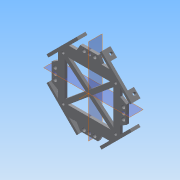
# Autodesk Inventor part: fix_board
Saved by Autodesk Inventor 2015 (Build 190159000, 159)
## iProperties
Created: 2015-06-18
Part Number: fix_board
Material: Générique
Document SubType Name: Modeling
Designer: Gregwar
Density: 1 g/cm^3
Appearance: Par défaut
Author: Gregwar
Autodesk Inventor part; units mm, degrees
ref_plane "YZ Plane" through (0, 0, 0) normal (1, 0, 0) x (0, 1, 0)
ref_plane "XZ Plane" through (0, 0, 0) normal (0, 1, 0) x (-1, 0, 0)
ref_plane "XY Plane" through (0, 0, 0) normal (0, 0, 1) x (1, 0, 0)
sketch "Esquisse1" plane through (0, 0, 0) normal (0, 1, 0) x (-1, 0, 0)
  line L0 (35, 35) -> (35, 14)
  line L1 (35, 14) -> (42, 10)
  line L2 (42, 10) -> (42, 0)
  line L3 (35, 35) -> (0, 0)
  line L4 (42, 0) -> (0, 0) construction
  line L5 (35, -35) -> (35, -14)
  line L6 (35, -14) -> (42, -10)
  line L7 (42, -10) -> (42, 0)
  line L8 (35, -35) -> (0, 0)
  line L9 (38.5, -12) -> (38.5, 12) construction
  circle A0 centre (38.5, 0) radius 2.15
  circle A1 centre (38.5, 6) radius 2.15
  circle A2 centre (38.5, -6) radius 2.15
  dimension "d0" = 90
  dimension "d1" = 70
  dimension "d4" = 6
  dimension "d11" = 6
  dimension "d16" = 4.3
  dimension "d17" = 20
  dimension "d18" = 4
  dimension "d19" = 7
  constraints: 20 end point, 3 centre point, 3 midpoint, 3 symmetric about line, 3 vertical, 1 horizontal, 1 parallel, 4 other
  measures "d0" angle of L3 L8
  measures "d1" distance of L0.start L5.start
  measures "d4" distance of A0.centre A1.centre
  measures "d11" distance of A0.centre A2.centre
  measures "d16" diameter of A0
  measures "d17" distance of L1.end L6.end
  measures "d18" vertical distance of L1.end L0.end
  measures "d19" distance between parallel lines of L5 L7
extrude "Extrusion1" add sketch "Esquisse1" along normal blind 3
pattern_circular "Réseau circulaire1" count 4 over 360 about axis through (0, 0, 0) along (0, 1, 0) of "Extrusion1"
sketch "Esquisse2" plane through (0, 3, 0) normal (0, 1, 0) x (1, 0, 0)
  circle A0 centre (0, -38.5) radius 2.15 construction
  circle A1 centre (6, -38.5) radius 2.15 construction
  circle A2 centre (-6, -38.5) radius 2.15 construction
  circle A3 centre (38.5, -6) radius 2.15 construction
  circle A4 centre (38.5, 6) radius 2.15 construction
  circle A5 centre (38.5, 0) radius 2.15 construction
  circle A6 centre (6, 38.5) radius 2.15 construction
  circle A7 centre (-6, 38.5) radius 2.15 construction
  circle A8 centre (0, 38.5) radius 2.15 construction
  circle A9 centre (-38.5, 6) radius 2.15 construction
  circle A10 centre (-38.5, -6) radius 2.15 construction
  circle A11 centre (-38.5, 0) radius 2.15 construction
  line L0 (-35, 35) -> (-35, 14) construction
  line L1 (-35, 14) -> (-42, 10) construction
  line L2 (-42, 10) -> (-42, -10) construction
  line L3 (-42, -10) -> (-35, -14) construction
  line L4 (-35, -14) -> (-35, -35) construction
  line L5 (-35, -35) -> (-14, -35) construction
  line L6 (-14, -35) -> (-10, -42) construction
  line L7 (-10, -42) -> (10, -42) construction
  line L8 (10, -42) -> (14, -35) construction
  line L9 (14, -35) -> (35, -35) construction
  line L10 (35, -35) -> (35, -14) construction
  line L11 (35, -14) -> (42, -10) construction
  line L12 (42, -10) -> (42, 10) construction
  line L13 (42, 10) -> (35, 14) construction
  line L14 (35, 14) -> (35, 35) construction
  line L15 (35, 35) -> (14, 35) construction
  line L16 (14, 35) -> (10, 42) construction
  line L17 (10, 42) -> (-10, 42) construction
  line L18 (-10, 42) -> (-14, 35) construction
  line L19 (-14, 35) -> (-35, 35) construction
  line L20 (32.5, -27.5) -> (-32.5, -27.5) construction
  line L21 (-32.5, -27.5) -> (-32.5, 27.5) construction
  line L22 (-32.5, 27.5) -> (32.5, 27.5) construction
  line L23 (32.5, 27.5) -> (32.5, -27.5) construction
  line L24 (32.5, -27.5) -> (-32.5, 27.5) construction
  line L25 (-32.5, -27.5) -> (32.5, 27.5) construction
  line L26 (29.5, -24.9615) -> (-29.5, -24.9615) construction
  line L27 (-29.5, -24.9615) -> (-29.5, 24.9615) construction
  line L28 (-29.5, 24.9615) -> (29.5, 24.9615) construction
  line L29 (29.5, 24.9615) -> (29.5, -24.9615) construction
  line L30 (29.5, -24.9615) -> (-29.5, 24.9615) construction
  line L31 (-29.5, -24.9615) -> (29.5, 24.9615) construction
  line L32 (27.5, -23.2692) -> (-27.5, -23.2692)
  line L33 (-27.5, -23.2692) -> (-27.5, 23.2692)
  line L34 (-27.5, 23.2692) -> (27.5, 23.2692)
  line L35 (27.5, 23.2692) -> (27.5, -23.2692)
  line L36 (27.5, -23.2692) -> (-27.5, 23.2692) construction
  line L37 (-27.5, -23.2692) -> (27.5, 23.2692) construction
  circle A12 centre (-29.5, -24.9615) radius 1.65
  circle A13 centre (29.5, -24.9615) radius 1.65
  circle A14 centre (29.5, 24.9615) radius 1.65
  circle A15 centre (-29.5, 24.9615) radius 1.65
  point P0 (0, 0)
  dimension "d25" = 65
  dimension "d26" = 55
  dimension "d27" = 3
  dimension "d28" = 2
  dimension "d29" = 3.3
  constraints: 36 end point, 6 midpoint, 6 parallel, 4 centre point, 4 coincident, 3 equal radius, 3 horizontal, 3 perpendicular, 2 point on line
  measures "d25" distance of L21.end L22.end
  measures "d26" distance of L20.end L21.end
  measures "d27" distance between parallel lines of L21 L27
  measures "d28" distance between parallel lines of L33 L27
  measures "d29" diameter of A12
extrude "Extrusion2" cut sketch "Esquisse2" against normal through all
chamfer "Chanfrein1" distance 8 angle 45 4 edges at (35, 1.5, -35) (-35, 1.5, -35) (-35, 1.5, 35) (35, 1.5, 35)
sketch "Esquisse3" plane through (0, 0, 0) normal (0, -1, 0) x (1, 0, 0)
  circle A0 centre (-29.5, -24.9615) radius 1.65 projected
  circle A1 centre (29.5, 24.9615) radius 1.65 projected
  circle A2 centre (-29.5, 24.9615) radius 1.65 projected
  circle A3 centre (29.5, -24.9615) radius 1.65 projected
  line L0 (27.5, 23.2692) -> (27.5, -23.2692) projected
  line L1 (27.5, -23.2692) -> (-27.5, -23.2692) projected
  line L2 (-27.5, -23.2692) -> (-27.5, 23.2692) projected
  line L3 (-27.5, 23.2692) -> (27.5, 23.2692) projected
  circle A4 centre (0, 38.5) radius 2.15 projected
  circle A5 centre (6, 38.5) radius 2.15 projected
  circle A6 centre (-6, 38.5) radius 2.15 projected
  circle A7 centre (38.5, 6) radius 2.15 projected
  circle A8 centre (38.5, -6) radius 2.15 projected
  circle A9 centre (38.5, 0) radius 2.15 projected
  circle A10 centre (6, -38.5) radius 2.15 projected
  circle A11 centre (-6, -38.5) radius 2.15 projected
  circle A12 centre (0, -38.5) radius 2.15 projected
  circle A13 centre (-38.5, -6) radius 2.15 projected
  circle A14 centre (-38.5, 6) radius 2.15 projected
  circle A15 centre (-38.5, 0) radius 2.15 projected
  line L4 (27, 35) -> (35, 27) projected
  line L5 (27, 35) -> (14, 35) projected
  line L6 (14, 35) -> (10, 42) projected
  line L7 (10, 42) -> (-10, 42) projected
  line L8 (-10, 42) -> (-14, 35) projected
  line L9 (-14, 35) -> (-27, 35) projected
  line L10 (-35, 27) -> (-27, 35) projected
  line L11 (-35, 27) -> (-35, 14) projected
  line L12 (-35, 14) -> (-42, 10) projected
  line L13 (-42, 10) -> (-42, -10) projected
  line L14 (-42, -10) -> (-35, -14) projected
  line L15 (-35, -14) -> (-35, -27) projected
  line L16 (-27, -35) -> (-35, -27) projected
  line L17 (-27, -35) -> (-14, -35) projected
  line L18 (-14, -35) -> (-10, -42) projected
  line L19 (-10, -42) -> (10, -42) projected
  line L20 (10, -42) -> (14, -35) projected
  line L21 (14, -35) -> (27, -35) projected
  line L22 (35, -27) -> (27, -35) projected
  line L23 (35, -27) -> (35, -14) projected
  line L24 (35, -14) -> (42, -10) projected
  line L25 (42, -10) -> (42, 10) projected
  line L26 (42, 10) -> (35, 14) projected
  line L27 (35, 14) -> (35, 27) projected
  line L28 (-47.9706, 14.0294) -> (-14.0294, 47.9706)
  line L29 (-14.0294, 47.9706) -> (-11.9081, 45.8492)
  line L30 (-11.9081, 45.8492) -> (-45.8492, 11.9081)
  line L31 (-45.8492, 11.9081) -> (-47.9706, 14.0294)
  point P0 (0, 0)
  point P1 (-31, 31)
  dimension "d35" = 48
  dimension "d36" = 3
  constraints: 8 end point, 2 midpoint, 2 perpendicular, 1 collinear, 1 parallel
  measures "d35" distance of L28.start L28.end
  measures "d36" distance of L28.end L29.end
extrude "Extrusion3" add sketch "Esquisse3" against normal blind 10 contours L30 L11 L10 L9 | L9 L28 L29 L30 | L30 L31 L28 L11
sketch "Esquisse4" plane through (-14.0294, 0, 47.9706) normal (-0.7071068, 0, 0.7071068) x (0.7071068, 0, 0.7071068)
  line L0 (0, 0) -> (-48, 0) projected
  line L1 (0, 0) -> (0, 10) projected
  line L2 (-48, 10) -> (0, 10) projected
  line L3 (-48, 0) -> (-48, 10) projected
  line L4 (-48, 0) -> (-48, 10) construction
  line L5 (-48, 7) -> (0, 7) construction
  line L6 (0, 0) -> (0, 10) construction
  circle A0 centre (-42.5, 7) radius 1.75
  line L7 (0, 10) -> (-48, 10) construction
  line L8 (-24, 10) -> (-24, 0) construction
  circle A1 centre (-5.5, 7) radius 1.75
  dimension "d41" = 10
  dimension "d42" = 3
  dimension "d43" = 37
  dimension "d44" = 3.5
  constraints: 4 end point, 3 point on line, 2 centre point, 1 horizontal, 1 midpoint, 1 symmetric about line, 1 vertical, 1 other
  measures "d41" distance between parallel lines of L0 L2
  measures "d42" distance between parallel lines of L5 L2
  measures "d43" distance of A0.centre A1.centre
  measures "d44" diameter of A0
extrude "Extrusion4" cut sketch "Esquisse4" against normal through all contours A0 | A1
ref_plane "Plan de construction1" through (0, 0, 14) normal (-1, 0, 0) x (0, 0, 1)
ref_plane "Plan de construction2" through (14, 0, 0) normal (0, 0, -1) x (-1, 0, 0)
sketch "Esquisse6" plane through (-14.0294, 0, 47.9706) normal (-0.7071068, 0, 0.7071068) x (0.7071068, 0, 0.7071068)
  line L0 (-15.3431, 3) -> (-9.1508, 3) projected
  circle A0 centre (-5.5, 7) radius 1.75 projected
  circle A1 centre (-42.5, 7) radius 1.75 projected
  line L1 (0, 0) -> (-48, 0) projected
  line L2 (0, 0) -> (0, 10) projected
  line L3 (-48, 10) -> (0, 10) projected
  line L4 (-48, 0) -> (-48, 10) projected
  line L5 (-10.5, 10) -> (-37.5, 10)
  line L6 (-37.5, 10) -> (-37.5, 3)
  line L7 (-37.5, 3) -> (-10.5, 3)
  line L8 (-10.5, 3) -> (-10.5, 10)
  point P0 (-24, 0)
  point P1 (-24, 10)
  dimension "d51" = 27
  dimension "d63" = 3
  constraints: 8 end point, 2 midpoint, 2 parallel, 1 horizontal, 1 perpendicular
  measures "d51" distance of L6.end L7.end
  measures "d63" distance between parallel lines of L7 L1
extrude "Extrusion5" cut sketch "Esquisse6" against normal through all contours L7 L6 L3 L8 L0
pattern_circular "Réseau circulaire4" count 4 over 360 about axis through (0, 0, 0) along (0, -1, 0) of "Extrusion5", "Extrusion4", "Extrusion3"
sketch "Esquisse8" plane through (0, 0, 0) normal (0, -1, 0) x (1, 0, 0)
  circle A0 centre (-29.5, -24.9615) radius 1.65 construction
  circle A1 centre (29.5, 24.9615) radius 1.65 construction
  circle A2 centre (-29.5, 24.9615) radius 1.65 construction
  circle A3 centre (29.5, -24.9615) radius 1.65 construction
  line L0 (27.5, 23.2692) -> (27.5, -23.2692) construction
  line L1 (27.5, -23.2692) -> (-27.5, -23.2692) construction
  line L2 (-27.5, -23.2692) -> (-27.5, 23.2692) construction
  line L3 (-27.5, 23.2692) -> (27.5, 23.2692) construction
  circle A4 centre (0, 38.5) radius 2.15 construction
  circle A5 centre (6, 38.5) radius 2.15 construction
  circle A6 centre (-6, 38.5) radius 2.15 construction
  circle A7 centre (38.5, 6) radius 2.15 construction
  circle A8 centre (38.5, -6) radius 2.15 construction
  circle A9 centre (38.5, 0) radius 2.15 construction
  circle A10 centre (6, -38.5) radius 2.15 construction
  circle A11 centre (-6, -38.5) radius 2.15 construction
  circle A12 centre (0, -38.5) radius 2.15 construction
  circle A13 centre (-38.5, -6) radius 2.15 construction
  circle A14 centre (-38.5, 6) radius 2.15 construction
  circle A15 centre (-38.5, 0) radius 2.15 construction
  line L4 (22.7574, 35) -> (14, 35) construction
  line L5 (14, 35) -> (10, 42) construction
  line L6 (10, 42) -> (-10, 42) construction
  line L7 (-10, 42) -> (-14, 35) construction
  line L8 (-14, 35) -> (-22.7574, 35) construction
  line L9 (-22.7574, 35) -> (-11.9081, 45.8492) construction
  line L10 (-11.9081, 45.8492) -> (-14.0294, 47.9706) construction
  line L11 (-14.0294, 47.9706) -> (-47.9706, 14.0294) construction
  line L12 (-47.9706, 14.0294) -> (-45.8492, 11.9081) construction
  line L13 (-45.8492, 11.9081) -> (-35, 22.7574) construction
  line L14 (-35, 22.7574) -> (-35, 14) construction
  line L15 (-35, 14) -> (-42, 10) construction
  line L16 (-42, 10) -> (-42, -10) construction
  line L17 (-42, -10) -> (-35, -14) construction
  line L18 (-35, -14) -> (-35, -22.7574) construction
  line L19 (-35, -22.7574) -> (-45.8492, -11.9081) construction
  line L20 (-45.8492, -11.9081) -> (-47.9706, -14.0294) construction
  line L21 (-47.9706, -14.0294) -> (-14.0294, -47.9706) construction
  line L22 (-14.0294, -47.9706) -> (-11.9081, -45.8492) construction
  line L23 (-11.9081, -45.8492) -> (-22.7574, -35) construction
  line L24 (-22.7574, -35) -> (-14, -35) construction
  line L25 (-14, -35) -> (-10, -42) construction
  line L26 (-10, -42) -> (10, -42) construction
  line L27 (10, -42) -> (14, -35) construction
  line L28 (14, -35) -> (22.7574, -35) construction
  line L29 (22.7574, -35) -> (11.9081, -45.8492) construction
  line L30 (11.9081, -45.8492) -> (14.0294, -47.9706) construction
  line L31 (14.0294, -47.9706) -> (47.9706, -14.0294) construction
  line L32 (47.9706, -14.0294) -> (45.8492, -11.9081) construction
  line L33 (45.8492, -11.9081) -> (35, -22.7574) construction
  line L34 (35, -22.7574) -> (35, -14) construction
  line L35 (35, -14) -> (42, -10) construction
  line L36 (42, -10) -> (42, 10) construction
  line L37 (42, 10) -> (35, 14) construction
  line L38 (35, 14) -> (35, 22.7574) construction
  line L39 (35, 22.7574) -> (45.8492, 11.9081) construction
  line L40 (45.8492, 11.9081) -> (47.9706, 14.0294) construction
  line L41 (47.9706, 14.0294) -> (14.0294, 47.9706) construction
  line L42 (14.0294, 47.9706) -> (11.9081, 45.8492) construction
  line L43 (11.9081, 45.8492) -> (22.7574, 35) construction
  line L44 (-27.5, 23.2692) -> (-23.9503, 23.2692)
  line L45 (27.5, 23.2692) -> (-27.5, 23.2692) projected
  line L46 (-23.9503, 23.2692) -> (27.5, -19.7195)
  line L47 (27.5, -23.2692) -> (27.5, 23.2692) projected
  line L48 (27.5, -19.7195) -> (27.5, -23.2692)
  line L49 (27.5, -23.2692) -> (23.9503, -23.2692)
  line L50 (-27.5, -23.2692) -> (27.5, -23.2692) projected
  line L51 (23.9503, -23.2692) -> (-27.5, 19.7195)
  line L52 (-27.5, 23.2692) -> (-27.5, -23.2692) projected
  line L53 (-27.5, 19.7195) -> (-27.5, 23.2692)
  line L54 (0, 23.2692) -> (0, -23.2692) construction
  circle A16 centre (29.5, -24.9615) radius 1.65 construction
  circle A17 centre (-29.5, 24.9615) radius 1.65 construction
  circle A18 centre (29.5, 24.9615) radius 1.65 construction
  circle A19 centre (-29.5, -24.9615) radius 1.65 construction
  line L55 (-27.5, 23.2692) -> (-27.5, -23.2692) construction
  line L56 (-27.5, -23.2692) -> (27.5, -23.2692) construction
  line L57 (27.5, -23.2692) -> (27.5, 23.2692) construction
  line L58 (27.5, 23.2692) -> (-27.5, 23.2692) construction
  circle A20 centre (-38.5, 6) radius 2.15 construction
  circle A21 centre (-38.5, -6) radius 2.15 construction
  circle A22 centre (-38.5, 0) radius 2.15 construction
  circle A23 centre (38.5, -6) radius 2.15 construction
  circle A24 centre (38.5, 6) radius 2.15 construction
  circle A25 centre (38.5, 0) radius 2.15 construction
  line L59 (-22.7574, 35) -> (-14, 35) construction
  line L60 (14, 35) -> (22.7574, 35) construction
  line L61 (47.9706, 14.0294) -> (45.8492, 11.9081) construction
  line L62 (45.8492, 11.9081) -> (35, 22.7574) construction
  line L63 (35, 22.7574) -> (35, 14) construction
  line L64 (35, 14) -> (42, 10) construction
  line L65 (42, 10) -> (42, -10) construction
  line L66 (42, -10) -> (35, -14) construction
  line L67 (35, -14) -> (35, -22.7574) construction
  line L68 (35, -22.7574) -> (45.8492, -11.9081) construction
  line L69 (45.8492, -11.9081) -> (47.9706, -14.0294) construction
  line L70 (22.7574, -35) -> (14, -35) construction
  line L71 (-14, -35) -> (-22.7574, -35) construction
  line L72 (-47.9706, -14.0294) -> (-45.8492, -11.9081) construction
  line L73 (-45.8492, -11.9081) -> (-35, -22.7574) construction
  line L74 (-35, -22.7574) -> (-35, -14) construction
  line L75 (-35, -14) -> (-42, -10) construction
  line L76 (-42, -10) -> (-42, 10) construction
  line L77 (-42, 10) -> (-35, 14) construction
  line L78 (-35, 14) -> (-35, 22.7574) construction
  line L79 (-35, 22.7574) -> (-45.8492, 11.9081) construction
  line L80 (-45.8492, 11.9081) -> (-47.9706, 14.0294) construction
  line L81 (27.5, 23.2692) -> (23.9503, 23.2692)
  line L82 (-27.5, 23.2692) -> (27.5, 23.2692)
  line L83 (23.9503, 23.2692) -> (-27.5, -19.7195)
  line L84 (-27.5, -23.2692) -> (-27.5, 23.2692)
  line L85 (-27.5, -19.7195) -> (-27.5, -23.2692)
  line L86 (-27.5, -23.2692) -> (-23.9503, -23.2692)
  line L87 (27.5, -23.2692) -> (-27.5, -23.2692)
  line L88 (-23.9503, -23.2692) -> (27.5, 19.7195)
  line L89 (27.5, 23.2692) -> (27.5, -23.2692)
  line L90 (27.5, 19.7195) -> (27.5, 23.2692)
  point P0 (0, 0)
  point P1 (-6, 38.5)
  point P2 (6, 38.5)
  dimension "d60" = 5
  constraints: 86 end point, 48 symmetric about line, 10 centre point, 8 point on line, 2 collinear, 2 equal length, 2 midpoint, 1 parallel, 10 other
  measures "d60" distance between parallel lines of L51 L46
extrude "Extrusion6" add sketch "Esquisse8" against normal blind 3 contours L44 L46 L83 L51 L52 | L45 L47 L88 L46 L83 | L46 L88 L51 L83 | L51 L88 L50 L52 L83 | L46 L47 L49 L51 L88
